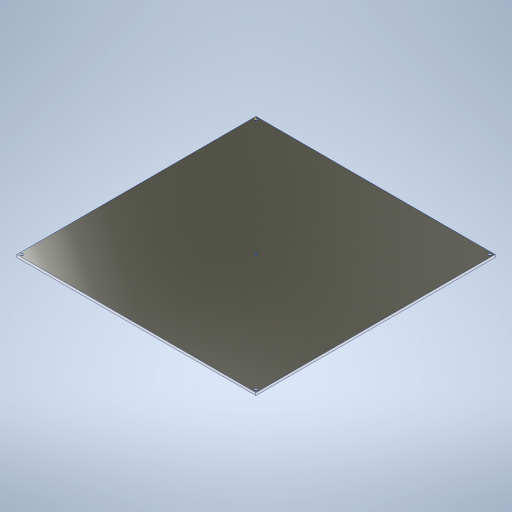
# Autodesk Inventor part: Base
Saved by Autodesk Inventor 2024 (Build 280153000, 153)
## iProperties
Created: 2024-05-05
Part Number: Base
Material: Alumínio 6061
Document SubType Name: Modeling
Designer: mathe
Density: 2.7 g/cm^3
Appearance: Alumínio - Plano
Author: mathe
Autodesk Inventor part; units mm, degrees
ref_plane "YZ Plane" through (0, 0, 0) normal (1, 0, 0) x (0, 1, 0)
ref_plane "XZ Plane" through (0, 0, 0) normal (0, 1, 0) x (-1, 0, 0)
ref_plane "XY Plane" through (0, 0, 0) normal (0, 0, 1) x (1, 0, 0)
sketch "Esboço1" plane through (0, 0, 0) normal (0, 1, 0) x (-1, 0, 0)
  line L0 (10.8534, 1800.0739) -> (-1804.1466, 1800.0739)
  line L1 (-1804.1466, 1800.0739) -> (-1804.1466, -14.9261)
  line L2 (-1804.1466, -14.9261) -> (10.8534, -14.9261)
  line L3 (10.8534, -14.9261) -> (10.8534, 1800.0739)
  point P0 (0, 0)
  dimension "d0" = 1815
  dimension "d1" = 1815
  constraints: 8 end point, 2 parallel, 1 horizontal, 1 perpendicular
  measures "d0" distance of L2.end L1.end
  measures "d1" distance between parallel lines of L2 L0
extrude "Extrusão1" add sketch "Esboço1" along normal blind 20
sketch "Esboço2" plane through (0, 20, 0) normal (0, 1, 0) x (1, 0, 0)
  circle A0 centre (896.6466, -892.5739) radius 11
  line L0 (1804.1466, -1800.0739) -> (1804.1466, 14.9261) projected
  line L1 (-10.8534, -1800.0739) -> (1804.1466, -1800.0739) projected
  circle A1 centre (9.1466, -5.0739) radius 10
  line L2 (1804.1466, 14.9261) -> (-10.8534, 14.9261) projected
  line L3 (-10.8534, 14.9261) -> (-10.8534, -1800.0739) projected
  circle A2 centre (1784.1466, -5.0739) radius 10
  circle A3 centre (1784.1466, -1780.0739) radius 10
  circle A4 centre (9.1466, -1780.0739) radius 10
  point P0 (0, 0)
  dimension "d4" = 22
  dimension "d5" = 907.5
  dimension "d6" = 907.5
  dimension "d29" = 20
  dimension "d30" = 20
  dimension "d31" = 20
  dimension "d32" = 20
  dimension "d33" = 20
  dimension "d34" = 20
  dimension "d35" = 20
  dimension "d36" = 20
  dimension "d37" = 20
  dimension "d38" = 20
  dimension "d39" = 20
  dimension "d40" = 20
  constraints: 5 centre point
  measures "d4" diameter of A0
  measures "d5" distance from line of L0 A0.centre
  measures "d6" distance from line of L1 A0.centre
  measures "d29" diameter of A1
  measures "d30" distance from line of L2 A1.centre
  measures "d31" distance from line of L3 A1.centre
  measures "d32" diameter of A2
  measures "d33" diameter of A3
  measures "d34" diameter of A4
  measures "d35" distance from line of L1 A4.centre
  measures "d36" distance from line of L3 A4.centre
  measures "d37" distance from line of L0 A2.centre
  measures "d38" distance from line of L2 A2.centre
  measures "d39" distance from line of L0 A3.centre
  measures "d40" distance from line of L1 A3.centre
hole "Furo1" at (1784.1466, 20, 1780.0739) at (1784.1466, 20, 5.0739) at (9.1466, 20, 5.0739) at (9.1466, 20, 1780.0739) direction (0, -1, 0) diameter 20 depth 10
sketch "Esboço3" plane through (0, 20, 0) normal (0, 1, 0) x (1, 0, 0)
  point P0 (0, 0)
sketch "Esboço4" plane through (0, 20, 0) normal (0, 1, 0) x (1, 0, 0)
  circle A0 centre (896.6466, -892.5739) radius 11
  line L0 (-10.8534, 14.9261) -> (-10.8534, -1800.0739) projected
  line L1 (1804.1466, 14.9261) -> (-10.8534, 14.9261) projected
  point P0 (0, 0)
  dimension "d41" = 22
  dimension "d42" = 907.5
  dimension "d43" = 907.5
  constraints: 1 centre point
  measures "d41" diameter of A0
  measures "d42" distance from line of L0 A0.centre
  measures "d43" distance from line of L1 A0.centre
hole "Furo2" at (896.6466, 20, 892.5739) direction (0, -1, 0) diameter 20 depth 15 counterbore diameter 22 counterbore depth 8
